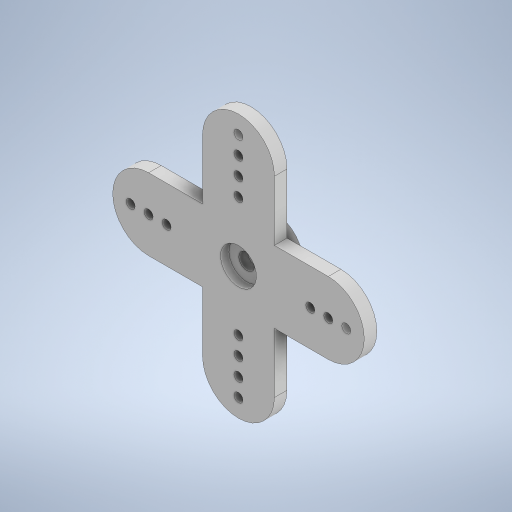
# Autodesk Inventor part: Standar Servo Horn - Red
Saved by Autodesk Inventor 2023 (Build 270158000, 158)
## iProperties
Created: 2023-09-03
Part Number: Standar Servo Horn - Red
Material: Generic
Document SubType Name: Modeling
Designer: Nate
Density: 1 g/cm^3
Appearance: Default
Author: Nate
Autodesk Inventor part; units mm, degrees
ref_plane "YZ Plane" through (0, 0, 0) normal (1, 0, 0) x (0, 1, 0)
ref_plane "XZ Plane" through (0, 0, 0) normal (0, 1, 0) x (-1, 0, 0)
ref_plane "XY Plane" through (0, 0, 0) normal (0, 0, 1) x (1, 0, 0)
sketch "Sketch1" plane through (0, 0, 0) normal (1, 0, 0) x (0, 1, 0)
  line L0 (0, 0) -> (6, 0)
  line L1 (6, 0) -> (6, -2.85)
  line L2 (6, -2.85) -> (0, -2.85)
  line L3 (0, -2.85) -> (0, 0)
  line L4 (0, 0) -> (3, 0)
  line L5 (3, 0) -> (3, -1.4)
  line L6 (3, -1.4) -> (0, -1.4)
  line L7 (0, -1.4) -> (0, 0)
  line L8 (0, -1.4) -> (1.35, -1.4)
  line L9 (1.35, -1.4) -> (1.35, -2.85)
  line L10 (1.35, -2.85) -> (0, -2.85)
  line L11 (0, -2.85) -> (0, -1.4)
  line L12 (0, -2.85) -> (5, -2.85)
  line L13 (5, -2.85) -> (5, -5.85)
  line L14 (5, -5.85) -> (0, -5.85)
  line L15 (0, -5.85) -> (0, -2.85)
  line L16 (0, -2.85) -> (2.75, -2.85)
  line L17 (2.75, -2.85) -> (2.75, -5.85)
  line L18 (2.75, -5.85) -> (0, -5.85)
  line L19 (0, -5.85) -> (0, -2.85)
  point P0 (1.5, 0)
  point P1 (1.5, -1.4)
  dimension "d0" = 6
  dimension "d1" = 2.85
  dimension "d2" = 3
  dimension "d3" = 1.4
  dimension "d4" = 1.35
  dimension "d5" = 1.45
  dimension "d6" = 5
  dimension "d7" = 3
  dimension "d8" = 2.75
  dimension "d9" = 3
  constraints: 40 end point, 10 parallel, 5 horizontal, 5 perpendicular, 2 midpoint
  measures "d0" distance of L1.end L2.end
  measures "d1" distance of L0.end L1.end
  measures "d2" distance of L5.end L6.end
  measures "d3" distance of point (1.5, 0) point (1.5, -1.4)
  measures "d4" distance of L9.end L10.end
  measures "d5" distance of L8.end L9.end
  measures "d6" distance of L13.end L14.end
  measures "d7" distance between parallel lines of L14 L2
  measures "d8" distance of L17.end L18.end
  measures "d9" distance of L16.end L17.end
revolve "Revolution1" add sketch "Sketch1" angle 360 about axis through (0, 0, -2.85) along (0, 0, 1) contours L0 L1 L2 L9 L6 L5 | L13 L14 L17 L2
sketch "Sketch2" plane through (0, 0, 0) normal (0, 0, 1) x (1, 0, 0)
  point P0 (0, 0)
sketch "Sketch3" plane through (0, 0, 0) normal (0, 0, 1) x (1, 0, 0)
  circle A0 centre (0, 16) radius 6
  circle A1 centre (-15, 0) radius 6
  circle A2 centre (0, -16) radius 6
  circle A3 centre (15, 0) radius 6
  line L0 (-6, 16) -> (-6, -16)
  line L1 (6, 16) -> (6, -16)
  line L2 (-15, 6) -> (15, 6)
  line L3 (-15, -6) -> (15, -6)
  circle A4 centre (0, 10) radius 0.75
  circle A5 centre (0, 13) radius 0.75
  circle A6 centre (0, 16) radius 0.75
  circle A7 centre (0, 19) radius 0.75
  circle A8 centre (0, -19) radius 0.75
  circle A9 centre (0, -16) radius 0.75
  circle A10 centre (0, -13) radius 0.75
  circle A11 centre (0, -10) radius 0.75
  circle A12 centre (-12, 0) radius 0.75
  circle A13 centre (-15, 0) radius 0.75
  circle A14 centre (-18, 0) radius 0.75
  circle A15 centre (12, 0) radius 0.75
  circle A16 centre (15, 0) radius 0.75
  circle A17 centre (18, 0) radius 0.75
  point P0 (0, 0)
  point P1 (-6, 6)
  point P2 (-6, -6)
  point P3 (6, -6)
  point P4 (6, 6)
  dimension "d11" = 12
  dimension "d12" = 16
  dimension "d13" = 12
  dimension "d14" = 15
  dimension "d15" = 12
  dimension "d16" = 16
  dimension "d17" = 12
  dimension "d18" = 15
  dimension "d19" = 1.5
  dimension "d20" = 1.5
  dimension "d21" = 1.5
  dimension "d22" = 1.5
  dimension "d23" = 10
  dimension "d24" = 13
  dimension "d25" = 16
  dimension "d26" = 19
  dimension "d27" = 1.5
  dimension "d28" = 1.5
  dimension "d29" = 1.5
  dimension "d30" = 1.5
  dimension "d31" = 10
  dimension "d32" = 13
  dimension "d33" = 16
  dimension "d34" = 19
  dimension "d35" = 1.5
  dimension "d36" = 1.5
  dimension "d37" = 1.5
  dimension "d38" = 12
  dimension "d39" = 15
  dimension "d40" = 18
  dimension "d41" = 1.5
  dimension "d42" = 1.5
  dimension "d43" = 1.5
  dimension "d44" = 18
  dimension "d45" = 15
  dimension "d46" = 12
  constraints: 18 centre point, 9 point on circle, 8 end point, 4 tangent, 1 parallel, 1 perpendicular, 1 vertical
  measures "d11" diameter of A0
  measures "d12" distance of A0.centre point (0, 0)
  measures "d13" diameter of A1
  measures "d14" distance of point (0, 0) A1.centre
  measures "d15" diameter of A2
  measures "d16" distance of point (0, 0) A2.centre
  measures "d17" diameter of A3
  measures "d18" distance of A3.centre point (0, 0)
  measures "d19" diameter of A4
  measures "d20" diameter of A5
  measures "d21" diameter of A6
  measures "d22" diameter of A7
  measures "d23" distance of point (0, 0) A4.centre
  measures "d24" distance of point (0, 0) A5.centre
  measures "d25" distance of point (0, 0) A6.centre
  measures "d26" distance of point (0, 0) A7.centre
  measures "d27" diameter of A8
  measures "d28" diameter of A9
  measures "d29" diameter of A10
  measures "d30" diameter of A11
  measures "d31" distance of point (0, 0) A11.centre
  measures "d32" distance of point (0, 0) A10.centre
  measures "d33" distance of point (0, 0) A9.centre
  measures "d34" distance of point (0, 0) A8.centre
  measures "d35" diameter of A12
  measures "d36" diameter of A13
  measures "d37" diameter of A14
  measures "d38" distance of point (0, 0) A12.centre
  measures "d39" distance of point (0, 0) A13.centre
  measures "d40" distance of point (0, 0) A14.centre
  measures "d41" diameter of A15
  measures "d42" diameter of A16
  measures "d43" diameter of A17
  measures "d44" distance of point (0, 0) A17.centre
  measures "d45" distance of point (0, 0) A16.centre
  measures "d46" distance of point (0, 0) A15.centre
extrude "Extrusion1" add sketch "Sketch3" against normal blind 2.1 contours A0 A4 | L1 L2 L0 A0 A4 | L2 A3 L3 L1 | L1 L3 L0 L2 | L0 L3 A1 L2 | L1 A2 A11 L0 L3 | A3 | A1 | A2 A11 picked at (-2.215, 14.0731) picked at (-2.215, -14.0731)
revolve "Revolution2" cut sketch "Sketch1" angle 360 about axis through (0, 0, -2.85) along (0, 0, 1) contours L0 L5 L6 L3 | L6 L9 L2 L3 | L2 L17 L14 L15
sketch "Sketch4" plane through (0, 0, -2.85) normal (0, 0, -1) x (-1, 0, 0)
  circle A0 centre (0, 0) radius 6
  circle A1 centre (0, 0) radius 1.35 projected
  circle A2 centre (0, 0) radius 5
  constraints: 2 centre point, 2 coincident
extrude "Extrusion2" add sketch "Sketch4" along normal blind 0.15 contours A0
body "Solid1"
